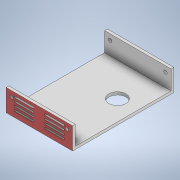
# Autodesk Inventor part: Caja2
Saved by Autodesk Inventor 2021 (Build 250183000, 183)
## iProperties
Created: 2021-02-22
Part Number: Caja2
Material: Generic
Document SubType Name: Modeling
Designer: deuts
Density: 1 g/cm^3
Appearance: Default
Author: deuts
Autodesk Inventor part; units mm, degrees
ref_plane "YZ Plane" through (0, 0, 0) normal (1, 0, 0) x (0, 1, 0)
ref_plane "XZ Plane" through (0, 0, 0) normal (0, 1, 0) x (-1, 0, 0)
ref_plane "XY Plane" through (0, 0, 0) normal (0, 0, 1) x (1, 0, 0)
sketch "Sketch1" plane through (0, 0, 0) normal (0, 1, 0) x (-1, 0, 0)
  line L0 (-60, 91.5) -> (60, 91.5)
  line L1 (60, 91.5) -> (60, -91.5)
  line L2 (60, -91.5) -> (-60, -91.5)
  line L3 (-60, -91.5) -> (-60, 91.5)
  line L4 (-60, 91.5) -> (60, -91.5) construction
  line L5 (60, 91.5) -> (-60, -91.5) construction
  point P0 (0, 0)
  dimension "d0" = 120
  dimension "d1" = 183
  constraints: 12 end point, 2 midpoint, 2 parallel, 1 horizontal, 1 perpendicular
  measures "d0" distance of L1.end L2.end
  measures "d1" distance of L0.end L1.end
extrude "Extrusion1" add sketch "Sketch1" along normal blind 5
sketch "Sketch2" plane through (0, 5, 0) normal (0, 1, 0) x (1, 0, 0)
  line L0 (-60, 91.5) -> (-60, -91.5) projected
  line L1 (60, -91.5) -> (60, 91.5) projected
  line L2 (-60, -91.5) -> (60, -91.5)
  line L3 (60, -91.5) -> (60, -86.5)
  line L4 (60, -86.5) -> (-60, -86.5)
  line L5 (-60, -86.5) -> (-60, -91.5)
  point P0 (0, 0)
  dimension "d4" = 5
  constraints: 8 end point, 2 parallel, 1 horizontal, 1 perpendicular, 1 point on line
  measures "d4" distance of L3.end L2.end
extrude "Extrusion2" add sketch "Sketch2" along normal blind 34.5
sketch "Sketch3" plane through (0, 5, 0) normal (0, 1, 0) x (1, 0, 0)
  line L0 (60, 91.5) -> (-60, 91.5) projected
  line L1 (60, -91.5) -> (60, 91.5) projected
  line L2 (-60, 91.5) -> (60, 91.5)
  line L3 (60, 91.5) -> (60, 86.5)
  line L4 (60, 86.5) -> (-60, 86.5)
  line L5 (-60, 86.5) -> (-60, 91.5)
  point P0 (0, 0)
  dimension "d7" = 5
  constraints: 8 end point, 2 parallel, 1 horizontal, 1 perpendicular, 1 point on line
  measures "d7" distance of L2.end L3.end
extrude "Extrusion3" add sketch "Sketch3" along normal blind 34.5
sketch "Sketch4" plane through (0, 0, 0) normal (0, -1, 0) x (1, 0, 0)
  circle A0 centre (23.62, -25.9) radius 15.35
  line L0 (-60, 91.5) -> (60, 91.5) projected
  line L1 (-60, -91.5) -> (-60, 91.5) projected
  point P0 (0, 0)
  dimension "d11" = 30.7
  dimension "d14" = 117.4
  dimension "d15" = 83.62
  constraints: 1 centre point
  measures "d11" diameter of A0
  measures "d14" distance from line of L0 A0.centre
  measures "d15" distance from line of L1 A0.centre
extrude "Extrusion4" cut sketch "Sketch4" against normal through all
sketch "Sketch5" plane through (-60, 0, 91.5) normal (0, 0, 1) x (1, 0, 0)
  line L0 (104, 10) -> (71, 10)
  line L1 (70, 11) -> (70, 12)
  line L2 (71, 13) -> (104, 13)
  line L3 (105, 12) -> (105, 11)
  line L4 (120, 0) -> (120, 39.5) projected
  line L5 (0, 0) -> (120, 0) projected
  arc A0 (104, 10) -> (105, 11) centre (104, 11) ccw
  arc A1 (105, 12) -> (104, 13) centre (104, 12) ccw
  arc A2 (70, 11) -> (71, 10) centre (71, 11) ccw
  arc A3 (71, 13) -> (70, 12) centre (71, 12) ccw
  point P0 (60, 0)
  point P1 (105, 10)
  point P2 (70, 13)
  point P3 (70, 10)
  point P4 (105, 13)
  dimension "d16" = 15
  dimension "d17" = 10
  dimension "d18" = 3
  dimension "d19" = 35
  dimension "d22" = 1
  constraints: 8 end point, 8 point on circle, 8 point on line, 8 tangent, 4 centre point, 3 equal radius, 2 parallel, 1 horizontal, 1 perpendicular
  measures "d16" distance between parallel lines of L4 L3
  measures "d17" distance from line of L5 point (105, 10)
  measures "d18" distance of point (70, 10) point (70, 13)
  measures "d19" distance of point (70, 13) point (105, 13)
  measures "d22" radius of A0
extrude "Extrusion5" cut sketch "Sketch5" against normal blind 5
mirror "Mirror1" about plane through (0, 0, 0) normal (1, 0, 0) of "Extrusion5"
pattern_linear "Rectangular Pattern1" count 4 spacing 7 along (0, 1, 0) of "Extrusion5", "Mirror1", "Extrusion4"
sketch "Sketch6" plane through (-60, 0, 91.5) normal (0, 0, 1) x (1, 0, 0)
  circle A0 centre (110, 29.5) radius 3
  line L0 (120, 0) -> (120, 39.5) projected
  line L1 (0, 39.5) -> (120, 39.5) projected
  point P0 (60, 0)
  dimension "d26" = 6
  dimension "d27" = 10
  dimension "d28" = 10
  constraints: 1 centre point
  measures "d26" diameter of A0
  measures "d27" distance from line of L0 A0.centre
  measures "d28" distance from line of L1 A0.centre
extrude "Extrusion6" cut sketch "Sketch6" against normal through all
mirror "Mirror2" about plane through (0, 0, 0) normal (1, 0, 0) of "Extrusion6"
body "Solid1"
